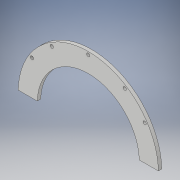
# Autodesk Inventor part: BearingGuard2
Saved by Autodesk Inventor 2018 (Build 220112000, 112)
## iProperties
Created: 2019-02-07
Part Number: BearingGuard2
Material: Generic
Document SubType Name: Modeling
Designer: anirudh
Density: 1 g/cm^3
Appearance: Default
Author: anirudh
Autodesk Inventor part; units mm, degrees
ref_plane "YZ Plane" through (0, 0, 0) normal (1, 0, 0) x (0, 1, 0)
ref_plane "XZ Plane" through (0, 0, 0) normal (0, 1, 0) x (-1, 0, 0)
ref_plane "XY Plane" through (0, 0, 0) normal (0, 0, 1) x (1, 0, 0)
sketch "Sketch1" plane through (0, 0, 0) normal (0, 0, 1) x (1, 0, 0)
  line L0 (0, 0) -> (101.8286, 0)
  line L1 (0, 0) -> (20.5964, 0) construction
  line L2 (101.8286, 0) -> (127.0177, 0) construction
  line L3 (0, 0) -> (-4.7595, 4.7595)
  line L4 (101.8286, 0) -> (106.5881, 4.7595)
  arc A0 (106.5881, 4.7595) -> (-4.7595, 4.7595) centre (50.9143, -50.5077) ccw
  circle A1 centre (10.0759, 12.4968) radius 1.85
  circle A2 centre (50.9143, 24.5745) radius 1.85
  circle A3 centre (91.7527, 12.4968) radius 1.85
  dimension "d7" = 3.7
  dimension "d8" = 3.7
  dimension "d9" = 3.7
  constraints: 10 end point, 4 centre point, 3 horizontal, 2 point on circle
  measures "d7" diameter of A1
  measures "d8" diameter of A2
  measures "d9" diameter of A3
extrude "Extrusion1" add sketch "Sketch1" along normal blind 3.81
sketch "Sketch2" plane through (0, 0, 3.81) normal (0, 0, 1) x (1, 0, 0)
  line L0 (0, 0) -> (101.8286, 0) projected
  line L1 (0, 0) -> (101.8286, 0)
  line L2 (50.9143, 6.604) -> (7.5245, 6.604)
  line L3 (50.9143, 6.604) -> (94.3041, 6.604)
  arc A0 (101.8286, 0) -> (94.3041, 6.604) centre (50.9143, -50.4221) ccw
  arc A1 (7.5245, 6.604) -> (0, 0) centre (50.9143, -50.4221) ccw
  constraints: 6 end point, 4 point on circle, 2 centre point, 1 collinear, 1 horizontal, 1 point on line
extrude "Extrusion2" cut sketch "Sketch2" against normal blind 3.81
fillet "Fillet1" radius 3.175 2 edges at (7.5245, 6.604, 1.905) (94.3041, 6.604, 1.905)
sketch "Sketch3" plane through (0, 0, 3.81) normal (0, 0, 1) x (1, 0, 0)
  arc A0 (106.5881, 4.7595) -> (-4.7595, 4.7595) centre (50.9143, -50.5077) ccw projected
  circle A1 centre (50.9143, -50.5077) radius 78.4477
  circle A2 centre (50.9143, -50.5077) radius 57.1117
  line L0 (8.6086, 6.604) -> (93.22, 6.604) projected
  circle A3 centre (50.9143, 24.5745) radius 1.85 projected
  circle A4 centre (10.0759, 12.4968) radius 1.85 projected
  circle A5 centre (91.7527, 12.4968) radius 1.85 projected
  circle A6 centre (-12.0871, -9.6645) radius 1.85
  circle A7 centre (-24.168, -50.5077) radius 1.85
  circle A8 centre (-12.0871, -91.3509) radius 1.85
  circle A9 centre (10.0759, -113.5123) radius 1.85
  circle A10 centre (50.9143, -125.59) radius 1.85
  circle A11 centre (91.7527, -113.5123) radius 1.85
  circle A12 centre (113.9157, -91.3509) radius 1.85
  circle A13 centre (125.9966, -50.5077) radius 1.85
  circle A14 centre (113.9157, -9.6645) radius 1.85
  point P0 (0, 0)
  dimension "d19" = 3.7
  dimension "d20" = 3.7
  dimension "d21" = 3.7
  dimension "d22" = 3.7
  dimension "d23" = 3.7
  dimension "d24" = 3.7
  dimension "d25" = 3.7
  dimension "d26" = 3.7
  dimension "d27" = 3.7
  constraints: 11 centre point, 2 coincident, 1 tangent
  measures "d19" diameter of A6
  measures "d20" diameter of A7
  measures "d21" diameter of A8
  measures "d22" diameter of A9
  measures "d23" diameter of A10
  measures "d24" diameter of A11
  measures "d25" diameter of A12
  measures "d26" diameter of A13
  measures "d27" diameter of A14
extrude "Extrusion3" add sketch "Sketch3" against normal blind 3.81
sketch "Sketch4" plane through (50.9143, -50.5077, 3.81) normal (0, 0, 1) x (1, 0, 0)
  circle A0 centre (-75.0823, 0) radius 1.85 projected
  line L0 (-75.0823, 1.85) -> (-55.8129, 1.85)
  line L1 (-75.0823, 1.85) -> (-78.4259, 1.85)
  line L2 (-78.4259, 1.85) -> (78.4259, 1.85)
  arc A1 (-78.4259, 1.85) -> (78.4259, 1.85) centre (0, 0) ccw
  point P0 (-50.9143, 50.5077)
  constraints: 6 end point, 3 horizontal, 2 point on circle, 1 centre point, 1 vertical alignment, 1 other
extrude "Extrusion4" cut sketch "Sketch4" against normal blind 3.81
body "Solid1"
